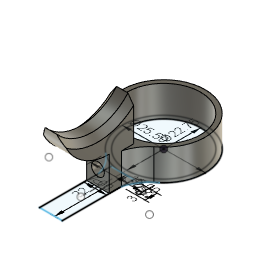
NeutronaWandClaw (Autodesk Fusion 360 design; units mm, degrees)
Autodesk Fusion 360 part; units mm, degrees
sketch "Top Sketch" plane through (0, 0, 0) normal (0, 0, 1) x (1, 0, 0)
  circle A0 centre (0, 0) radius 12.75
  circle A1 centre (0, 0) radius 11.375
  line L0 (3.5, -12.7849) -> (3.5, -34.7849)
  line L1 (3.5, -34.7849) -> (-3.5, -34.7849)
  line L2 (-3.5, -34.7849) -> (-3.5, -12.7849)
  line L3 (0, 0) -> (0, -25.5697) construction
  line L4 (-3.5, -12.7849) -> (3.5, -12.7849)
  arc A2 (8.2587, -9.7137) -> (3.5, -16.5349) centre (15.3325, -19.7192) ccw
  arc A3 (-3.5, -16.5349) -> (-7.7413, -10.1309) centre (-15.5185, -19.8881) ccw
  dimension "d1" = 25.5
  dimension "d2" = 22.75
  dimension "d4" = 22
  dimension "d5" = 7
  dimension "d20" = 90
  dimension "d30" = 16
  dimension "d31" = 3.75
  constraint coincident A0.centre A1.centre
  constraint vertical L0
  constraint perpendicular L0 L1
  constraint perpendicular L1 L2
  constraint vertical L3
  constraint coincident A0 A2.start
  constraint coincident L0 A2.end
  constraint coincident A0 A3.end
  constraint coincident L2 A3.start
  constraint horizontal A2.end A3.start
  constraint midpoint L3 L4
  measures "d1" diameter of A0
  measures "d2" diameter of A1
  measures "d4" distance of L0.start L0.end
  measures "d5" distance of L0 L2
  measures "d20" angle of L0 L4
  measures "d30" horizontal distance of A2.start A3.end
  measures "d31" distance of L0.start A2.end
extrude "Ring Extrude" add sketch "Top Sketch" along normal blind 9.5 contours A0 A2 | A0 L0 L2 L4 A2 A3 | A0 A2
extrude "Claw Extrude" add sketch "Top Sketch" along normal blind 22.25 contours L0 L1 L2 L4
sketch "Side Claw Sketch" plane through (3.5, 0, 0) normal (1, 0, 0) x (0, 1, 0)
  line L0 (-12.7849, 22.25) -> (-34.7849, 22.25)
  line L1 (-34.7849, 22.25) -> (-34.7849, 0)
  line L2 (-34.7849, 0) -> (-16.5349, 0)
  line L3 (-20.2849, 0) -> (-20.2849, 10.5)
  line L4 (-11.5398, 10.5) -> (-20.2849, 10.5) construction
  arc A0 (-34.7849, 22.25) -> (-12.7849, 22.25) centre (-23.7849, 31.85) ccw
  line L5 (-12.7849, 9.5) -> (-12.7849, 22.25)
  line L6 (-20.2849, 10.5) -> (-29.7849, 10.5) construction
  line L7 (-29.7849, 10.5) -> (-29.7849, 22.25) construction
  line L8 (-29.7849, 10.5) -> (-29.7849, 0) construction
  arc A1 (-34.7849, 22.25) -> (-20.2849, 10.5) centre (-20.2849, 25.3218) ccw
  line L9 (-16.5349, 0) -> (-16.5349, 9.5)
  line L10 (-16.5349, 9.5) -> (-12.7849, 9.5)
  point P0 (-23.7849, 17.25)
  point P1 (-23.7849, 22.25)
  dimension "d21" = 10.5
  dimension "d22" = 7.5
  dimension "d25" = 5
  dimension "d26" = 9.5
  constraint coincident L2 L3.start
  constraint perpendicular L2 L3
  constraint perpendicular L3 L4
  constraint coincident L0.start A0.end
  constraint coincident L0.end L1.start
  constraint midpoint A0 P0
  constraint midpoint L0 P1
  constraint perpendicular L3 L6
  constraint coincident L0 L7.end
  constraint perpendicular L0 L7
  constraint coincident L2 L8.end
  constraint perpendicular L2 L8
  constraint tangent L6 A1
  measures "d21" distance of L3.start L3.end
  measures "d22" distance of L3 L5
  measures "d25" distance of P0 P1
  measures "d26" distance of L3.end L6.end
extrude "Second Claw Extrude" cut sketch "Side Claw Sketch" against normal blind 10 contours L0 A0 | L1 L2 L3 A1
sketch "Screw Hole Sketch" plane through (0, -20.2849, 0) normal (0, -1, 0) x (1, 0, 0)
  line L0 (-3.5, 10.5) -> (-3.5, 0)
  line L1 (-3.5, 0) -> (3.5, 0)
  line L2 (3.5, 0) -> (3.5, 10.5)
  circle A0 centre (0, 4.75) radius 2.25
  line L3 (3.5, 10.5) -> (-3.5, 10.5)
  line L4 (3.5, 9.5) -> (7.3788, 9.5)
  dimension "d14" = 4.5
  dimension "d34" = 4.75
  constraint vertical origin A0.centre
  measures "d14" diameter of A0
  measures "d34" distance of A0.centre L4
chamfer "Claw Chamfer" distance 1.75 angle 45 2 edges at (3.5, -23.7849, 17.25) (-3.5, -23.7849, 17.25)
hole "Screw Hole" at (0, -20.2849, 4.75) direction (0, 1, 0) diameter 4 depth 15 tip angle 180
named bodies: "Wand Claw"
